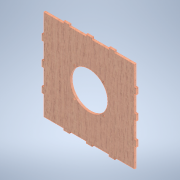
# Autodesk Inventor part: Верх
Saved by Autodesk Inventor 2021 (Build 250183000, 183)
## iProperties
Created: 2021-04-10
Part Number: Верх
Material: Типовые
Document SubType Name: Modeling
Designer: user
Density: 1 g/cm^3
Appearance: Белый дуб — натуральный — с умеренным глянцем
Author: user
Autodesk Inventor part; units mm, degrees
ref_plane "YZ Plane" through (0, 0, 0) normal (1, 0, 0) x (0, 1, 0)
ref_plane "XZ Plane" through (0, 0, 0) normal (0, 1, 0) x (-1, 0, 0)
ref_plane "XY Plane" through (0, 0, 0) normal (0, 0, 1) x (1, 0, 0)
sketch "Эскиз1" plane through (0, 0, 0) normal (0, 0, 1) x (1, 0, 0)
  circle A0 centre (0, 0) radius 30.75
  circle A1 centre (24, -24) radius 1.5
  circle A2 centre (24, 24) radius 1.5
  circle A3 centre (-24, 24) radius 1.5
  circle A4 centre (-24, -24) radius 1.5
  line L0 (-78, 42.5) -> (-75, 42.5)
  line L1 (-75, 32.5) -> (-78, 32.5)
  line L2 (-78, 32.5) -> (-78, 42.5)
  line L3 (-78, 5) -> (-75, 5)
  line L4 (-78, 0) -> (-78, 5)
  line L5 (-42.5, 78) -> (-32.5, 78)
  line L6 (-32.5, 78) -> (-32.5, 75)
  line L7 (-42.5, 75) -> (-42.5, 78)
  line L8 (-5, 78) -> (0, 78)
  line L9 (-5, 75) -> (-5, 78)
  line L10 (-5, 75) -> (-32.5, 75)
  line L11 (-42.5, 75) -> (-75, 75)
  line L12 (-75, 75) -> (-75, 42.5)
  line L13 (-75, 32.5) -> (-75, 5)
  line L14 (78, 42.5) -> (75, 42.5)
  line L15 (75, 32.5) -> (78, 32.5)
  line L16 (78, 32.5) -> (78, 42.5)
  line L17 (78, 5) -> (75, 5)
  line L18 (78, 0) -> (78, 5)
  line L19 (42.5, 78) -> (32.5, 78)
  line L20 (32.5, 78) -> (32.5, 75)
  line L21 (42.5, 75) -> (42.5, 78)
  line L22 (5, 78) -> (0, 78)
  line L23 (5, 75) -> (5, 78)
  line L24 (5, 75) -> (32.5, 75)
  line L25 (42.5, 75) -> (75, 75)
  line L26 (75, 5) -> (75, 32.5)
  line L27 (75, 75) -> (75, 42.5)
  line L28 (-78, -42.5) -> (-75, -42.5)
  line L29 (-75, -32.5) -> (-78, -32.5)
  line L30 (-78, -32.5) -> (-78, -42.5)
  line L31 (-78, -5) -> (-75, -5)
  line L32 (-78, 0) -> (-78, -5)
  line L33 (-42.5, -78) -> (-32.5, -78)
  line L34 (-32.5, -78) -> (-32.5, -75)
  line L35 (-42.5, -75) -> (-42.5, -78)
  line L36 (-5, -78) -> (0, -78)
  line L37 (-5, -75) -> (-5, -78)
  line L38 (-5, -75) -> (-32.5, -75)
  line L39 (-42.5, -75) -> (-75, -75)
  line L40 (-75, -5) -> (-75, -32.5)
  line L41 (-75, -75) -> (-75, -42.5)
  line L42 (75, -32.5) -> (78, -32.5)
  line L43 (75, -32.5) -> (75, -5)
  line L44 (78, -5) -> (75, -5)
  line L45 (78, 0) -> (78, -5)
  line L46 (78, -42.5) -> (75, -42.5)
  line L47 (78, -32.5) -> (78, -42.5)
  line L48 (5, -75) -> (32.5, -75)
  line L49 (5, -78) -> (0, -78)
  line L50 (5, -75) -> (5, -78)
  line L51 (75, -42.5) -> (75, -75)
  line L52 (42.5, -75) -> (75, -75)
  line L53 (32.5, -78) -> (32.5, -75)
  line L54 (42.5, -78) -> (32.5, -78)
  line L55 (42.5, -75) -> (42.5, -78)
  constraints: 112 end point, 6 horizontal, 5 centre point, 5 perpendicular, 4 coincident, 2 parallel
extrude "Выдавливание1" add sketch "Эскиз1" along normal blind 3
